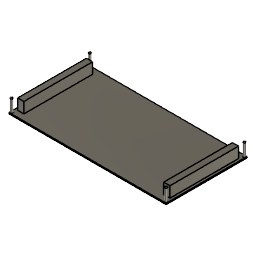
back_frame (Autodesk Fusion 360 design; units mm, degrees)
part number: 2026-05-15-00-05-07-772
Autodesk Fusion 360 part; units mm, degrees
sketch "Sketch1" plane through (0, 0, 0) normal (0, 0, 1) x (1, 0, 0)
  line L0 (-40, -50) -> (589, -50)
  line L1 (589, -50) -> (589, 274)
  line L2 (589, 274) -> (-40, 274)
  line L3 (-40, 274) -> (-40, -50)
  circle A0 centre (583.5, -44.5) radius 5
  circle A1 centre (583.5, 268.5) radius 5
  circle A2 centre (-34.5, 268.5) radius 5
  circle A3 centre (-34.5, -44.5) radius 5
  line L4 (-30, 250) -> (-5, 250)
  line L5 (-5, 250) -> (-5, -25)
  line L6 (-5, -25) -> (-30, -25)
  line L7 (-30, -25) -> (-30, 250)
  line L8 (579, 250) -> (554, 250)
  line L9 (554, 250) -> (554, -25)
  line L10 (554, -25) -> (579, -25)
  line L11 (579, -25) -> (579, 250)
  dimension "d1" = 629
  dimension "d2" = 324
  dimension "d3" = 10
  dimension "d4" = 5.5
  dimension "d5" = 5.5
  dimension "d6" = 10
  dimension "d7" = 5.5
  dimension "d8" = 5.5
  dimension "d9" = 10
  dimension "d10" = 5.5
  dimension "d11" = 5.5
  dimension "d12" = 10
  dimension "d13" = 5.5
  dimension "d14" = 5.5
  dimension "d15" = 10
  dimension "d16" = 559
  constraint horizontal L0
  constraint vertical L1
  constraint horizontal L2
  constraint vertical L3
  constraint horizontal L4
  constraint vertical L5
  constraint horizontal L6
  constraint vertical L7
  constraint horizontal L8
  constraint vertical L9
  constraint horizontal L10
  constraint vertical L11
  measures "d1" distance of L0.start L0.end
  measures "d2" distance of L0.start L2.end
  measures "d3" diameter of A0
  measures "d4" distance of L0 A0.centre
  measures "d5" distance of L1 A0.centre
  measures "d6" diameter of A1
  measures "d7" distance of L1 A1.centre
  measures "d8" distance of L2 A1.centre
  measures "d9" diameter of A2
  measures "d10" distance of L2 A2.centre
  measures "d11" distance of L3 A2.centre
  measures "d12" diameter of A3
  measures "d13" distance of L0 A3.centre
  measures "d14" distance of L3 A3.centre
  measures "d15" distance of L3 L7
  measures "d16" distance of L5 L9
extrude "Extrude1" add sketch "Sketch1" along normal blind 5
extrude "Extrude2" add sketch "Sketch1" along normal blind 48 contours L4 L5 L6 L7 | L8 L9 L10 L11
extrude "Extrude3" add sketch "Sketch1" along normal blind 55 contours A3
extrude "Extrude4" add sketch "Sketch1" along normal blind 55 contours A2
extrude "Extrude5" add sketch "Sketch1" along normal blind 55 contours A1
extrude "Extrude6" add sketch "Sketch1" along normal blind 55 contours A0
